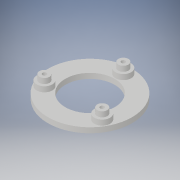
# Autodesk Inventor part: PlanetaryHolderBottom
Saved by Autodesk Inventor 2018.3 (Build 223284000, 284)
## iProperties
Created: 2018-07-08
Part Number: PlanetaryHolderBottom
Material: Generisch
Document SubType Name: Modeling
Designer: JochenAlt
Density: 1 g/cm^3
Appearance: Vorgabe
Author: JochenAlt
Autodesk Inventor part; units mm, degrees
ref_plane "YZ Plane" through (0, 0, 0) normal (1, 0, 0) x (0, 1, 0)
ref_plane "XZ Plane" through (0, 0, 0) normal (0, 1, 0) x (-1, 0, 0)
ref_plane "XY Plane" through (0, 0, 0) normal (0, 0, 1) x (1, 0, 0)
sketch "Skizze1" plane through (0, 0, 0) normal (0, 0, 1) x (1, 0, 0)
  line L0 (-33.894, 0) -> (33.894, 0) construction
  circle A0 centre (0, 0) radius 19.21 construction
  circle A1 centre (0, 19.21) radius 1.15
  circle A2 centre (16.6363, -9.605) radius 1.15
  circle A3 centre (-16.6363, -9.605) radius 1.15
  line L1 (0, 33.894) -> (0, -33.894) construction
  line L2 (0, 0) -> (-16.6363, -9.605) construction
  circle A4 centre (0, 0) radius 14.21
  circle A5 centre (0, 0) radius 24.21
  circle A6 centre (16.6363, -9.605) radius 2.9
  circle A7 centre (0, 19.21) radius 2.9
  circle A8 centre (-16.6363, -9.605) radius 2.9
  circle A9 centre (0, 19.21) radius 4.5
  circle A10 centre (16.6363, -9.605) radius 4.5
  circle A11 centre (-16.6363, -9.605) radius 4.5
  dimension "d0" = 38.42
  dimension "d1" = 2.3
  dimension "d2" = 30
  dimension "d3" = 5
  dimension "d4" = 5
  dimension "d21" = 5.8
  dimension "d27" = 9
  constraints: 12 centre point, 8 coincident, 6 equal radius, 4 point on circle, 2 end point, 1 other
  measures "d0" diameter of A0
  measures "d1" diameter of A1
  measures "d2" angle of L2 L0
  measures "d3" radial gap between concentric circles of A5 A0
  measures "d4" radial gap between concentric circles of A4 A0
  measures "d21" diameter of A7
  measures "d27" diameter of A9
extrude "Extrusion2" add sketch "Skizze1" along normal blind 3 contours A5 | A6 | A7 | A8 | A9 | A10 | A11
extrude "Extrusion4" add sketch "Skizze1" along normal blind 3 from surface at 3 contours A6 | A7 | A8 | A9 | A10 | A11
extrude "Extrusion5" add sketch "Skizze1" along normal blind 3 from surface at 6 contours A6 | A7 | A8
extrude "Extrusion6" cut sketch "Skizze1" along normal blind 2 contours A6 | A7 | A8
equation "\"d3\" = d4"
